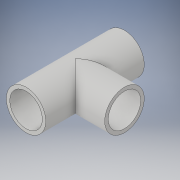
# Autodesk Inventor part: Tee 1 Inch
Saved by Autodesk Inventor 2018 (Build 220112000, 112)
## iProperties
Created: 2018-01-22
Part Number: Tee 1 Inch
Material: Generic
Document SubType Name: Modeling
Designer: owner
Density: 1 g/cm^3
Appearance: Default
Author: owner
Autodesk Inventor part; units mm, degrees
ref_plane "YZ Plane" through (0, 0, 0) normal (1, 0, 0) x (0, 1, 0)
ref_plane "XZ Plane" through (0, 0, 0) normal (0, 1, 0) x (-1, 0, 0)
ref_plane "XY Plane" through (0, 0, 0) normal (0, 0, 1) x (1, 0, 0)
sketch "Sketch1" plane through (0, 0, 0) normal (0, 0, 1) x (1, 0, 0)
  circle A0 centre (0, 0) radius 20.3835
  dimension "d0" = 40.767
  constraints: 1 centre point, 1 coincident
  measures "d0" diameter of A0
extrude "Extrusion1" add sketch "Sketch1" against normal blind 101.6
sketch "Sketch2" plane through (0, 0, 0) normal (0, 0, 1) x (1, 0, 0)
  circle A0 centre (0, 0) radius 20.3835 projected
  line L0 (20.3835, 0) -> (20.3835, 20.3835)
  constraints: 2 end point, 2 vertical, 1 horizontal alignment, 1 other
sketch "Sketch3" plane through (0, 0, -101.6) normal (0, 0, -1) x (-1, 0, 0)
  circle A0 centre (0, 0) radius 20.3835 projected
  line L0 (-20.3835, 0) -> (-20.3835, 20.3835)
  constraints: 2 end point, 2 vertical, 1 horizontal alignment, 1 other
ref_plane "Work Plane1" through (20.3835, 0, 0) normal (-1, 0, 0) x (0, 1, 0)
sketch "Sketch4" plane through (20.3835, 0, 0) normal (-1, 0, 0) x (0, 1, 0)
  line L0 (20.3835, 101.6) -> (-20.3835, 101.6) projected
  circle A0 centre (0, 50.8) radius 20.3835
  line L1 (-20.3835, 0) -> (-20.3835, 101.6) projected
  point P0 (0, 0)
  constraints: 1 centre point, 1 tangent
extrude "Extrusion2" add sketch "Sketch4" against normal blind 30.4165
extrude "Extrusion3" add sketch "Sketch4" along normal blind 20.3835
sketch "Sketch5" plane through (0, 0, 0) normal (0, 0, 1) x (1, 0, 0)
  circle A0 centre (0, 0) radius 16.7767
  dimension "d7" = 33.5534
  constraints: 1 centre point, 1 coincident
  measures "d7" diameter of A0
sketch "Sketch6" plane through (0, 0, 0) normal (0, 0, 1) x (1, 0, 0)
  circle A0 centre (0, 0) radius 12.7
  dimension "d8" = 25.4
  constraints: 1 centre point, 1 coincident
  measures "d8" diameter of A0
sketch "Sketch7" plane through (50.8, 0, -50.8) normal (1, 0, 0) x (0, 0, -1)
  circle A0 centre (0, 0) radius 16.7767
  point P0 (-50.8, 0)
  dimension "d9" = 33.5534
  constraints: 1 centre point
  measures "d9" diameter of A0
sketch "Sketch8" plane through (50.8, 0, -50.8) normal (1, 0, 0) x (0, 0, -1)
  circle A0 centre (0, 0) radius 12.7
  point P0 (-50.8, 0)
  dimension "d10" = 25.4
  constraints: 1 centre point
  measures "d10" diameter of A0
sketch "Sketch9" plane through (0, 0, -101.6) normal (0, 0, -1) x (-1, 0, 0)
  circle A0 centre (0, 0) radius 16.7767
  dimension "d11" = 33.5534
  constraints: 1 centre point, 1 coincident
  measures "d11" diameter of A0
extrude "Extrusion4" cut sketch "Sketch9" against normal blind 31.6992
extrude "Extrusion5" cut sketch "Sketch7" against normal blind 31.6992
extrude "Extrusion6" cut sketch "Sketch5" against normal blind 31.6992
extrude "Extrusion7" cut sketch "Sketch6" against normal blind 101.6
extrude "Extrusion8" cut sketch "Sketch8" against normal blind 50.8
body "Solid1"
